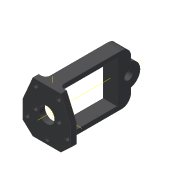
# Autodesk Inventor part: empty
Saved by Autodesk Inventor 2014 (Build 180170000, 170)
## iProperties
Created: 2015-04-13
Part Number: empty
Material: Generic
Document SubType Name: Modeling
Designer: Martin
Density: 1 g/cm^3
Appearance: Default
Author: Martin
Autodesk Inventor part; units mm, degrees
ref_plane "YZ Plane" through (0, 0, 0) normal (1, 0, 0) x (0, 1, 0)
ref_plane "XZ Plane" through (0, 0, 0) normal (0, 1, 0) x (-1, 0, 0)
ref_plane "XY Plane" through (0, 0, 0) normal (0, 0, 1) x (1, 0, 0)
sketch "sk_main" plane through (0, 0, 0) normal (1, 0, 0) x (0, 1, 0)
  line L0 (-10, 0) -> (42.5, 0) projected
  line L1 (0, -15.4) -> (0, 15.4) projected
  line L2 (25, -9) -> (0, -9)
  line L3 (0, -9) -> (0, 9)
  line L4 (0, 9) -> (25, 9)
  line L5 (25, 9) -> (25, -9)
  line L6 (25, -9) -> (0, 9) construction
  line L7 (0, -9) -> (25, 9) construction
  circle A0 centre (30, 0) radius 1.75
  circle A1 centre (30, 0) radius 5 construction
  line L8 (-2.5, 11) -> (31, 11)
  line L9 (31, 11) -> (31, 4.899)
  line L10 (31, -4.899) -> (31, -11)
  line L11 (31, -11) -> (-2.5, -11)
  line L12 (-2.5, -11) -> (-2.5, 11)
  arc A2 (31, -4.899) -> (31, 4.899) centre (30, 0) ccw
  line L13 (0, 11) -> (0, -11)
  point P0 (0, 0)
  point P1 (12.5, 0)
  dimension "d0" = 25
  dimension "d1" = 18
  dimension "d2" = 3.5
  dimension "d3" = 5
  dimension "d4" = 2
  dimension "d5" = 2.5
  dimension "d6" = 1
  constraints: 24 end point, 5 perpendicular, 5 point on line, 4 point on circle, 3 centre point, 3 collinear, 3 parallel, 2 midpoint, 2 tangent, 1 coincident, 1 concentric, 1 horizontal, 1 other
  measures "d0" distance of L3.end L4.end
  measures "d1" distance of L4.end L2.start
  measures "d2" diameter of A0
  measures "d3" distance from line of L5 A0.centre
  measures "d4" distance between parallel lines of L8 L4
  measures "d5" distance between parallel lines of L3 L12
  measures "d6" distance from line of A0.centre L9
extrude "ext_main_back" add sketch "sk_main" along normal mid plane 6 contours L5 L4 L1 L8 L9 A2 L0 A0 | L0 A0 A2 L10 L11 L1 L2 L5
extrude "ext_main_front" add sketch "sk_main" along normal mid plane 12.15 contours L12 L8 L1 L0 | L0 L1 L11 L12
sketch "sk_front" plane through (0, 0, 0) normal (0, 1, 0) x (-1, 0, 0)
  line L0 (0, -15.4) -> (0, 15.4) projected
  line L1 (8.505, 0) -> (-8.505, 0) projected
  circle A0 centre (0, 0) radius 3.4
  circle A1 centre (5.075, 0) radius 1
  circle A2 centre (-5.075, 0) radius 1
  circle A3 centre (0, 0) radius 8 construction
  circle A4 centre (0, -9) radius 8 construction
  circle A5 centre (0, -9) radius 1
  circle A6 centre (8.6494, -4.5) radius 1.75 construction
  circle A7 centre (-8.6494, -4.5) radius 1.75 construction
  line L2 (8.6494, -4.5) -> (-8.6494, -4.5) construction
  line L3 (-6.075, 11) -> (-6.075, -11) projected
  line L4 (6.075, -11) -> (6.075, 11) projected
  line L5 (10.3994, 1) -> (10.3994, -7)
  line L6 (10.3994, 1) -> (6.075, 11)
  line L7 (10.3994, -7) -> (6.075, -11)
  line L8 (-6.075, 11) -> (-10.3994, 1)
  line L9 (-10.3994, 1) -> (-10.3994, -7)
  line L10 (-10.3994, -7) -> (-6.075, -11)
  line L11 (6.075, -11) -> (-6.075, -11) projected
  circle A8 centre (-8.6494, -4.5) radius 1
  circle A9 centre (8.6494, -4.5) radius 1
  circle A10 centre (-5, 8.5) radius 1
  circle A11 centre (-5, 8.5) radius 2.25 construction
  line L12 (-5, 8.5) -> (5, 8.5) construction
  circle A12 centre (5, 8.5) radius 2.25 construction
  circle A13 centre (5, 8.5) radius 1
  point P0 (0, 8.5)
  dimension "d11" = 6.8
  dimension "d12" = 2
  dimension "d13" = 10.15
  dimension "d14" = 16
  dimension "d15" = 16
  dimension "d16" = 9
  dimension "d17" = 2
  dimension "d18" = 3.5
  dimension "d21" = 8
  dimension "d22" = 4
  dimension "d26" = 2
  dimension "d27" = 2
  dimension "d28" = 4.5
  dimension "d30" = 10
  dimension "d31" = 8.5
  constraints: 16 end point, 14 centre point, 8 coincident, 5 tangent, 4 equal radius, 4 point on line, 4 symmetric about line, 3 perpendicular, 2 parallel, 1 midpoint, 2 other
  measures "d11" diameter of A0
  measures "d12" diameter of A2
  measures "d13" distance of A2.centre A1.centre
  measures "d14" diameter of A3
  measures "d15" diameter of A4
  measures "d16" distance of A4.centre point (0, 0)
  measures "d17" diameter of A5
  measures "d18" diameter of A7
  measures "d21" distance of L5.start L5.end
  measures "d22" distance from line of L11 L5.end
  measures "d26" diameter of A9
  measures "d27" diameter of A10
  measures "d28" diameter of A11
  measures "d30" distance of L12.start L12.end
  measures "d31" distance between parallel lines of L1 L12
extrude "ext_front_tabs" add sketch "sk_front" against normal up to surface (2.5 mm away) contours L4 L6 L5 L7 | L10 L9 L8 L3 | A8 | A9
extrude "ext_cut_holesfront" cut sketch "sk_front" against normal through all contours A5 L0 | L0 A5 | A1 L1 | L1 A1 | A2 L1 | L1 A2 | A0 L1 L0 | L0 L1 A0 | L1 A0 L0 | L0 A0 L1 | A8 | A9 | A10 | A13
fillet "Fillet2" radius 2 2 edges at (3, 0, 10) (-3, 0, 10)
fillet "Fillet3" radius 3 2 edges at (3, 0, -10) (-3, 0, -10)
fillet "Fillet4" radius 4 2 edges at (0, 31, 11) (0, 31, -11)
extrude "ext_dowelfill" add sketch "sk_front" against normal blind 1.65 contours A5 L0 | L0 A5
equation "\"d2\" = screw_m3_bore_loose"
equation "\"d12\" = screw_m2_bore_selfthreading"
equation "\"d17\" = screw_m2_bore_selfthreading"
equation "\"d26\" = screw_m2_bore_selfthreading"
equation "\"d27\" = screw_m2_bore_selfthreading"
equation "\"d28\" = screw_m2_head_maxsize"
equation "\"screw_m3_bore_loose\" = 3.5"
equation "\"screw_m2_bore_selfthreading\" = 2"
equation "\"screw_m2_head_maxsize\" = 4.5"
body "Solid1"
